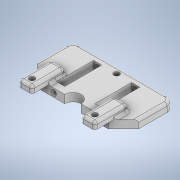
# Autodesk Inventor part: g2HEMount2
Saved by Autodesk Inventor 2020 (Build 240168000, 168)
## iProperties
Created: 2021-06-01
Part Number: g2HEMount2
Material: Generic
Document SubType Name: Modeling
Designer: PAB
Density: 1 g/cm^3
Appearance: Default
Author: PAB
Autodesk Inventor part; units mm, degrees
ref_plane "YZ Plane" through (0, 0, 0) normal (1, 0, 0) x (0, 1, 0)
ref_plane "XZ Plane" through (0, 0, 0) normal (0, 1, 0) x (-1, 0, 0)
ref_plane "XY Plane" through (0, 0, 0) normal (0, 0, 1) x (1, 0, 0)
sketch "Sketch1" plane through (0, 0, 0) normal (0, 1, 0) x (-1, 0, 0)
  line L0 (37, 37) -> (-37, 37)
  line L1 (-37, 37) -> (-37, -37)
  line L2 (-37, -37) -> (37, -37)
  line L3 (37, -37) -> (37, 37)
  point P0 (0, 0)
  dimension "d0" = 74
  dimension "d1" = 74
  constraints: 8 end point, 2 parallel, 1 horizontal, 1 perpendicular
  measures "d0" distance of L2.end L1.end
  measures "d1" distance of L1.end L0.end
extrude "Extrusion1" add sketch "Sketch1" along normal blind 6
fillet "Fillet1" radius 5 4 edges at (-37, 3, 37) (37, 3, 37) (37, 3, -37) (-37, 3, -37)
sketch "Sketch2" plane through (0, 6, 0) normal (0, 1, 0) x (1, 0, 0)
  line L0 (-37, 32) -> (-37, -32) projected
  line L1 (-37, 0) -> (37, 0)
  line L2 (37, -32) -> (37, 32) projected
  circle A0 centre (0, 0) radius 6
  line L3 (-37, 0) -> (37, 0)
  line L4 (37, 0) -> (37, 63.5)
  line L5 (37, 63.5) -> (-37, 63.5)
  line L6 (-37, 63.5) -> (-37, 0)
  line L7 (-6, 0) -> (-26, 0)
  line L8 (-26, 0) -> (-37, 11)
  line L9 (6, 0) -> (26, 0)
  line L10 (26, 0) -> (37, 11)
  circle A1 centre (32, 0) radius 2
  circle A2 centre (0, -32) radius 2
  circle A3 centre (-32, 0) radius 2
  circle A4 centre (0, 32) radius 2
  line L11 (-37, 0) -> (37, 0)
  line L12 (37, 0) -> (37, -38.1)
  line L13 (37, -38.1) -> (-37, -38.1)
  line L14 (-37, -38.1) -> (-37, 0)
  point P0 (-6, 0)
  dimension "d5" = 12
  dimension "d6" = 20
  dimension "d7" = 135
  dimension "d8" = 20
  dimension "d9" = 135
  dimension "d10" = 4
  dimension "d11" = 4
  dimension "d12" = 4
  dimension "d29" = 4
  constraints: 26 end point, 8 point on line, 5 centre point, 4 parallel, 2 horizontal, 2 midpoint, 2 perpendicular, 2 point on circle, 1 coincident
  measures "d5" diameter of A0
  measures "d6" distance of L7.start L7.end
  measures "d7" angle of L7 L8
  measures "d8" distance of L9.start L9.end
  measures "d9" angle of L10 L9
  measures "d10" diameter of A1
  measures "d11" diameter of A2
  measures "d12" diameter of A3
  measures "d29" diameter of A4
extrude "Extrusion2" cut sketch "Sketch2" against normal blind 10 contours L8 L1 A3 L0 | L1 A3 A0 A1 L2 L12 L13 L14 L0 | A3 L1 | L1 A3 | A0 L1 | L1 A0 | L2 L1 A1 L10 | A1 L1 | L1 A1 | A2 | A4
sketch "Sketch6" plane through (0, 6, 0) normal (0, 1, 0) x (1, 0, 0)
  line L0 (11, 5) -> (17, 5)
  line L1 (17, 5) -> (17, 32)
  line L2 (17, 32) -> (11, 32)
  line L3 (11, 32) -> (11, 5)
  line L4 (-11, 5) -> (-17, 5)
  line L5 (-17, 5) -> (-17, 32)
  line L6 (-17, 32) -> (-11, 32)
  line L7 (-11, 32) -> (-11, 5)
  point P0 (0, 0)
  dimension "d30" = 6
  dimension "d31" = 27
  dimension "d32" = 6
  dimension "d33" = 27
  constraints: 16 end point, 4 parallel, 2 horizontal, 2 perpendicular
  measures "d30" distance of L2.end L1.end
  measures "d31" distance of L1.end L0.end
  measures "d32" distance of L5.end L6.end
  measures "d33" distance of L4.end L5.end
extrude "Extrusion6" cut sketch "Sketch6" against normal blind 10
sketch "Sketch8" plane through (-26, 0, 0) normal (0, 0, 1) x (1, 0, 0)
  circle A0 centre (12, 3) radius 2
  circle A1 centre (40, 3) radius 2
  point P0 (26, 0)
  dimension "d44" = 4
  dimension "d45" = 4
  constraints: 2 centre point
  measures "d44" diameter of A0
  measures "d45" diameter of A1
extrude "Extrusion8" cut sketch "Sketch8" against normal blind 50
sketch "Sketch9" plane through (0, 6, 0) normal (0, 1, 0) x (1, 0, 0)
  circle A0 centre (-23, -7) radius 2
  circle A1 centre (23, -7) radius 2
  line L0 (-28, -12) -> (-18, -12)
  line L1 (-18, -12) -> (-18, 12)
  line L2 (-18, 12) -> (-28, 12)
  line L3 (-28, 12) -> (-28, -12)
  line L4 (18, -12) -> (28, -12)
  line L5 (28, -12) -> (28, 12)
  line L6 (28, 12) -> (18, 12)
  line L7 (18, 12) -> (18, -12)
  point P0 (0, 0)
  dimension "d48" = 4
  dimension "d49" = 4
  dimension "d50" = 10
  dimension "d51" = 24
  dimension "d52" = 10
  dimension "d53" = 24
  constraints: 16 end point, 4 parallel, 2 centre point, 2 horizontal, 2 perpendicular
  measures "d48" diameter of A0
  measures "d49" diameter of A1
  measures "d50" distance of L2.end L1.end
  measures "d51" distance of L1.end L0.end
  measures "d52" distance of L6.end L5.end
  measures "d53" distance of L5.end L4.end
extrude "Extrusion9" add sketch "Sketch9" along normal blind 5
fillet "Fillet3" radius 2 16 edges at (-23, 11, 12) (-18, 11, 0) (-28, 11, 0) (-23, 11, -12) (-28, 8.5, -12) (-18, 8.5, -12) (-28, 8.5, 12) (-18, 8.5, 12) (18, 11, 0) (23, 11, 12) (28, 11, 0) (23, 11, -12) (18, 8.5, 12) (28, 8.5, 12) (28, 8.5, -12) (18, 8.5, -12)
fillet "Fillet4" radius 2 15 edges at (18.5858, 6, -11.4142) (23, 6, -12) (27.4142, 6, -11.4142) (28, 6, -6) (18, 6, -5) (-27.4142, 6, -11.4142) (-23, 6, -12) (-18.5858, 6, -11.4142) (-18, 6, -5) (-28, 6, -6) (-35.5355, 6, -35.5355) (0, 6, -37) (35.5355, 6, -35.5355) (37, 6, -21.5) (-37, 6, -21.5)
body "Solid1"
